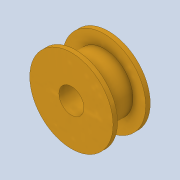
# Autodesk Inventor part: Roller
Saved by Autodesk Inventor 2020.4 (Build 244396000, 396)
## iProperties
Created: 2018-10-16
Part Number: Roller
Material: Brass, Soft Yellow, Welded
Document SubType Name: Modeling
Designer: victo
Mass: 0.396849 g
Surface Area: 1.59253 cm^2
Volume: 0.0466882 cm^3
Density: 8.5 g/cm^3
Appearance: Weld - Brass
Author: victo
Autodesk Inventor part; units mm, degrees
ref_plane "YZ Plane" through (0, 0, 0) normal (1, 0, 0) x (0, 1, 0)
ref_plane "XZ Plane" through (0, 0, 0) normal (0, 1, 0) x (-1, 0, 0)
ref_plane "XY Plane" through (0, 0, 0) normal (0, 0, 1) x (1, 0, 0)
sketch "Sketch1" plane through (0, 0, 0) normal (0, 0, 1) x (1, 0, 0)
  circle A0 centre (0, 0) radius 3.25
  dimension "d0" = 6.5
  constraints: 1 centre point, 1 coincident
  measures "d0" diameter of A0
extrude "Roller Base" add sketch "Sketch1" along normal mid plane 2.9
sketch "Sketch2" plane through (0, 0, 0) normal (0, 0, 1) x (1, 0, 0)
  circle A0 centre (0, 0) radius 0.975
  dimension "d3" = 1.95
  constraints: 1 centre point, 1 coincident
  measures "d3" diameter of A0
extrude "Roller Axis" cut sketch "Sketch2" along normal through all both and the other way through all
sketch "Sketch3" plane through (0, 0, 0) normal (0, 0, 1) x (1, 0, 0)
  circle A0 centre (0, 0) radius 0.975 projected
  circle A1 centre (0, 0) radius 3.25 projected
  circle A2 centre (0, 0) radius 2.25
  dimension "d6" = 4.5
  constraints: 1 centre point, 1 coincident
  measures "d6" diameter of A2
extrude "Roller Bar Fit" cut sketch "Sketch3" along normal mid plane 2.2 contours A1
body "Solid1"
